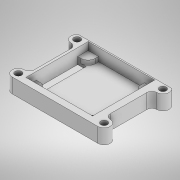
# Autodesk Inventor part: OledModBase
Saved by Autodesk Inventor 2021 (Build 250183000, 183)
## iProperties
Created: 2021-08-19
Part Number: OledModBase
Material: Generic
Document SubType Name: Modeling
Designer: perez
Density: 1 g/cm^3
Appearance: Default
Author: perez
Autodesk Inventor part; units mm, degrees
ref_plane "YZ Plane" through (0, 0, 0) normal (1, 0, 0) x (0, 1, 0)
ref_plane "XZ Plane" through (0, 0, 0) normal (0, 1, 0) x (-1, 0, 0)
ref_plane "XY Plane" through (0, 0, 0) normal (0, 0, 1) x (1, 0, 0)
sketch "Sketch1" plane through (0, 0, 0) normal (0, 1, 0) x (-1, 0, 0)
  line L0 (0, 0) -> (27, 0) construction
  line L1 (27, 0) -> (27, -25) construction
  line L2 (27, -25) -> (0, -25) construction
  line L3 (0, -25) -> (0, 0) construction
  line L4 (31, 2) -> (-4, 2)
  line L5 (-4, -27) -> (31, -27)
  line L6 (29, -22) -> (29, -3)
  line L7 (28, -4) -> (23.5, -4)
  line L8 (23.5, -4) -> (23.5, -21)
  line L9 (23.5, -21) -> (28, -21)
  line L10 (28, -21) -> (28, -4)
  arc A0 (31, -3) -> (31, 2) centre (31, -0.5) ccw
  arc A1 (31, -27) -> (31, -22) centre (31, -24.5) ccw
  arc A2 (-4, 2) -> (-4, -3) centre (-4, -0.5) ccw
  arc A3 (-4, -22) -> (-4, -27) centre (-4, -24.5) ccw
  line L11 (31, -3) -> (29, -3)
  line L12 (31, -22) -> (29, -22)
  line L13 (-4, -3) -> (-2, -3)
  line L14 (-4, -22) -> (-2, -22)
  line L15 (-2, -3) -> (-2, -22)
  circle A4 centre (31, -0.5) radius 1.35
  circle A5 centre (31, -24.5) radius 1.35
  circle A6 centre (-4, -0.5) radius 1.35
  circle A7 centre (-4, -24.5) radius 1.35
  point P0 (29, 2)
  point P1 (-2, -27)
  point P2 (-2, 2)
  point P3 (29, -27)
  dimension "d0" = 27
  dimension "d1" = 25
  dimension "d12" = 2
  dimension "d13" = 2
  dimension "d14" = 2
  dimension "d18" = 1
  dimension "d19" = 3.5
  dimension "d20" = 6
  dimension "d21" = 6
  dimension "d22" = 5
  dimension "d23" = 2.5
  dimension "d24" = 2
  dimension "d25" = 2.5
  dimension "d26" = 2
  dimension "d27" = 5
  dimension "d28" = 5
  dimension "d29" = 5
  dimension "d32" = 2.5
  dimension "d33" = 2.5
  dimension "d34" = 2.7
  dimension "d35" = 2.7
  dimension "d36" = 2.7
  dimension "d37" = 2.7
  constraints: 32 end point, 8 centre point, 8 point on circle, 7 parallel, 6 point on line, 5 perpendicular, 4 coincident, 3 horizontal, 3 tangent
  measures "d0" distance of L1.end L2.end
  measures "d1" distance of L0.end L1.end
  measures "d12" distance between parallel lines of L5 L2
  measures "d13" distance between parallel lines of L6 L1
  measures "d14" distance between parallel lines of L0 L4
  measures "d18" distance between parallel lines of L1 L10
  measures "d19" distance between parallel lines of L8 L1
  measures "d20" distance between parallel lines of L5 L9
  measures "d21" distance between parallel lines of L4 L7
  measures "d22" diameter of A0
  measures "d23" distance from line of L4 A0.centre
  measures "d24" distance from line of L6 A0.centre
  measures "d25" distance from line of L5 A1.centre
  measures "d26" distance from line of L6 A1.centre
  measures "d27" diameter of A1
  measures "d28" diameter of A2
  measures "d29" diameter of A3
  measures "d32" distance from line of L5 A3.centre
  measures "d33" distance from line of L4 A2.centre
  measures "d34" diameter of A4
  measures "d35" diameter of A5
  measures "d36" diameter of A6
  measures "d37" diameter of A7
extrude "Extrusion1" add sketch "Sketch1" against normal blind 1
sketch "Sketch2" plane through (0, 0, 0) normal (0, 1, 0) x (1, 0, 0)
  line L0 (-31, -2) -> (4, -2) projected
  arc A0 (4, -2) -> (4, 3) centre (4, 0.5) ccw projected
  line L1 (4, 3) -> (2, 3) projected
  line L2 (2, 3) -> (2, 22) projected
  line L3 (2, 22) -> (4, 22) projected
  arc A1 (4, 22) -> (4, 27) centre (4, 24.5) ccw projected
  line L4 (4, 27) -> (-31, 27) projected
  arc A2 (-31, 27) -> (-31, 22) centre (-31, 24.5) ccw projected
  line L5 (-31, 22) -> (-29, 22) projected
  line L6 (-29, 22) -> (-29, 3) projected
  line L7 (-29, 3) -> (-31, 3) projected
  arc A3 (-31, 3) -> (-31, -2) centre (-31, 0.5) ccw projected
  circle A4 centre (4, 24.5) radius 1.35 projected
  circle A5 centre (4, 0.5) radius 1.35 projected
  circle A6 centre (-31, 24.5) radius 1.35 projected
  circle A7 centre (-31, 0.5) radius 1.35 projected
  line L8 (-28, 4) -> (-28, 21) projected
  line L9 (-28, 21) -> (-23.5, 21) projected
  line L10 (-23.5, 21) -> (-23.5, 4) projected
  line L11 (-23.5, 4) -> (-28, 4) projected
  line L12 (-28, 26) -> (1, 26)
  line L13 (1, 26) -> (1, -1)
  line L14 (1, -1) -> (-28, -1)
  line L15 (-28, -1) -> (-28, 26)
  point P0 (0, 0)
  dimension "d38" = 1
  dimension "d39" = 1
  dimension "d40" = 1
  dimension "d41" = 1
  constraints: 8 end point, 2 parallel, 1 horizontal, 1 perpendicular
  measures "d38" distance between parallel lines of L2 L13
  measures "d39" distance between parallel lines of L12 L4
  measures "d40" distance between parallel lines of L6 L15
  measures "d41" distance between parallel lines of L0 L14
extrude "Extrusion2" add sketch "Sketch2" along normal blind 5
fillet "Fillet1" radius 2 4 edges at (2, 2, -3) (2, 2, -22) (-29, 2, -22) (-29, 2, -3)
sketch "Sketch4" plane through (0, 5, 0) normal (0, 1, 0) x (1, 0, 0)
  line L0 (-36.8851, 35.5263) -> (12.4576, 35.5263)
  line L1 (12.4576, 35.5263) -> (12.4576, 26.5)
  line L2 (12.4576, 26.5) -> (-36.8851, 26.5)
  line L3 (-36.8851, 26.5) -> (-36.8851, 35.5263)
  line L4 (4, 27) -> (-31, 27) projected
  point P0 (0, 0)
  dimension "d47" = 0.5
  constraints: 8 end point, 2 parallel, 1 horizontal, 1 perpendicular
  measures "d47" distance between parallel lines of L2 L4
extrude "Extrusion3" cut sketch "Sketch4" against normal blind 10
sketch "Sketch5" plane through (0, 0, 0) normal (0, 1, 0) x (1, 0, 0)
  line L0 (1, -1) -> (-28, -1) projected
  line L1 (-28, -1) -> (1, -1)
  line L2 (1, -1) -> (1, 0.6)
  line L3 (1, 0.6) -> (-28, 0.6)
  line L4 (-28, 0.6) -> (-28, -1)
  line L5 (1, 26) -> (1, -1) projected
  line L6 (1, 26) -> (-28, 26) projected
  line L7 (1, -1) -> (-0.8, -1)
  line L8 (-0.8, -1) -> (-0.8, 26)
  line L9 (-0.8, 26) -> (1, 26)
  line L10 (1, 26) -> (1, -1)
  point P0 (0, 0)
  point P1 (-0.8, 0.6)
  dimension "d50" = 1.6
  dimension "d57" = 1.8
  constraints: 16 end point, 4 parallel, 2 horizontal, 2 perpendicular, 1 point on line
  measures "d50" distance between parallel lines of L0 L3
  measures "d57" distance between parallel lines of L8 L5
extrude "Extrusion4" add sketch "Sketch5" along normal up to surface (5 mm away)
sketch "Sketch6" plane through (0, -1, 0) normal (0, -1, 0) x (1, 0, 0)
  line L0 (-23.5, -4) -> (-28, -4) projected
  line L1 (-28, -0.6) -> (-28, -26) projected
  line L2 (-23.5, -4) -> (-28, -4)
  line L3 (-28, -4) -> (-28, -8)
  line L4 (-28, -8) -> (-23.5, -8)
  line L5 (-23.5, -8) -> (-23.5, -4)
  line L6 (-28, -21) -> (-23.5, -21) projected
  line L7 (-23.5, -4) -> (-25.6, -4)
  line L8 (-25.6, -4) -> (-25.6, -21)
  line L9 (-25.6, -21) -> (-23.5, -21)
  line L10 (-23.5, -21) -> (-23.5, -4)
  point P0 (0, 0)
  point P1 (-25.6, -8)
  dimension "d53" = 4
  dimension "d54" = 2.4
  constraints: 16 end point, 4 parallel, 2 horizontal, 2 perpendicular, 2 point on line
  measures "d53" distance between parallel lines of L4 L0
  measures "d54" distance between parallel lines of L1 L8
extrude "Extrusion5" add sketch "Sketch6" against normal up to surface (1 mm away) contours L5 L4 L8 L0 | L8 L4 L1 L0 | L10 L6 L8 L4
sketch "Sketch7" plane through (0, 0, 0) normal (0, 1, 0) x (1, 0, 0)
  line L0 (-28, 0.6) -> (-0.8, 0.6) projected
  line L1 (-0.8, 0.6) -> (-5.1, 0.6)
  line L2 (-5.1, 0.6) -> (-5.1, 4.9)
  line L3 (-5.1, 4.9) -> (-0.8, 4.9)
  line L4 (-0.8, 4.9) -> (-0.8, 0.6)
  line L5 (-28, 0.6) -> (-23.7, 0.6)
  line L6 (-23.7, 0.6) -> (-23.7, 4.9)
  line L7 (-23.7, 4.9) -> (-28, 4.9)
  line L8 (-28, 4.9) -> (-28, 0.6)
  line L9 (-28, 26) -> (-0.8, 26) projected
  line L10 (-28, 26) -> (-23.7, 26)
  line L11 (-23.7, 26) -> (-23.7, 21.7)
  line L12 (-23.7, 21.7) -> (-28, 21.7)
  line L13 (-28, 21.7) -> (-28, 26)
  line L14 (-0.8, 26) -> (-5.1, 26)
  line L15 (-5.1, 26) -> (-5.1, 21.7)
  line L16 (-5.1, 21.7) -> (-0.8, 21.7)
  line L17 (-0.8, 21.7) -> (-0.8, 26)
  point P0 (0, 0)
  point P1 (-0.8, 26)
  dimension "d58" = 4.3
  dimension "d59" = 4.3
  dimension "d60" = 4.3
  dimension "d61" = 4.3
  dimension "d62" = 4.3
  dimension "d63" = 4.3
  constraints: 32 end point, 8 parallel, 4 horizontal, 4 perpendicular, 1 point on line
  measures "d58" distance of L2.end L3.end
  measures "d59" distance of L1.end L2.end
  measures "d60" distance of L7.end L6.end
  measures "d61" distance of L10.end L11.end
  measures "d62" distance of L16.end L15.end
  measures "d63" distance of L15.end L14.end
extrude "Extrusion6" add sketch "Sketch7" along normal blind 1.86
fillet "Fillet2" radius 3 4 edges at (-23.7, 0.93, -21.7) (-23.7, 0.93, -4.9) (-5.1, 0.93, -21.7) (-5.1, 0.93, -4.9)
sketch "Sketch8" plane through (0, 0, 0) normal (0, 1, 0) x (1, 0, 0)
  line L0 (-28, 21.7) -> (-28, 26) projected
  line L1 (-28, 21.7) -> (-24.5334, 21.7)
  line L2 (-24.5334, 21.7) -> (-24.5334, 4.9)
  line L3 (-24.5334, 4.9) -> (-28, 4.9)
  line L4 (-28, 4.9) -> (-28, 21.7)
  point P0 (0, 0)
  constraints: 8 end point, 2 parallel, 1 horizontal, 1 perpendicular
extrude "Extrusion7" cut sketch "Sketch8" against normal blind 10
equation "\"d13\" = d12"
equation "\"d14\" = d12"
equation "\"d15\" = d12"
body "Solid1"
